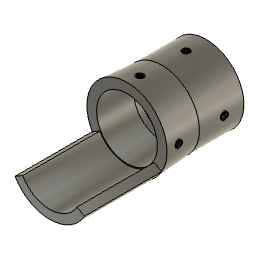
Microscope Holder v3 (Autodesk Fusion 360 design; units mm, degrees)
Autodesk Fusion 360 part; units mm, degrees
sketch "Sketch1" plane through (0, 0, 0) normal (0, 1, 0) x (1, 0, 0)
  circle A0 centre (0, 0) radius 14.5
  dimension "d1" = 29
  constraint coincident A0.centre origin
  measures "d1" diameter of A0
sketch "Sketch2" plane through (0, 0, 0) normal (0, 0, 1) x (1, 0, 0)
  line L0 (0, 0) -> (0, -18)
  dimension "d2" = 18
  constraint coincident L0.start origin
  constraint vertical L0
  measures "d2" distance of L0.start L0.end
sketch "Sketch3" plane through (0, 0, 0) normal (0, 1, 0) x (1, 0, 0)
  circle A0 through (15.75, 0, -18) (-7.875, 13.6399, -18) (-7.875, -13.6399, -18)
  dimension "d3" = 31.5
sketch "Sketch4" plane through (0, 0, 0) normal (0, 1, 0) x (1, 0, 0)
  circle A0 centre (0, 0) radius 19.5
  circle A1 centre (0, 0) radius 14.5
  dimension "d4" = 39
  dimension "d6" = 29
  constraint coincident A0.centre A1.centre
  constraint concentric A0 A1
  measures "d4" diameter of A0
  measures "d6" diameter of A1
sketch "Sketch5" plane through (0, -18, 0) normal (0, 1, 0) x (1, 0, 0)
  circle A0 centre (0, 0) radius 20.75
  circle A1 centre (0, 0) radius 15.75
  dimension "d5" = 41.5
  dimension "d7" = 31.5
  constraint coincident A0.centre A1.centre
  constraint concentric A0 A1
  measures "d5" diameter of A0
  measures "d7" diameter of A1
loft "Loft1" add profiles "Sketch4", "Sketch5" section 1 section 2
loft "Loft2" cut profiles "Sketch4", "Sketch5" section 1 contours A1 section 2 contours A1
extrude "Extrude1" add sketch "Sketch4" along normal blind 3
extrude "Extrude2" add 1 faces at (17.7067, 3, 1.6891) along direction (0, 1, 0) blind 0.05
sketch "Sketch6" plane through (0, 3.05, 0) normal (0, 1, 0) x (-1, 0, 0)
  circle A0 centre (0, 0) radius 14.5
  circle A1 centre (0, 0) radius 19.5
  circle A2 centre (0, 0) radius 10.775
  circle A3 centre (0, 0) radius 19.5
  dimension "d12" = 21.55
  constraint concentric A0 A2
  constraint concentric A0 A3
  measures "d12" diameter of A2
extrude "Extrude3" add sketch "Sketch6" along normal blind 20 contours A0 | A1 A3
sketch "Sketch7" plane through (0, 0, 0) normal (0, 0, 1) x (1, 0, 0)
  line L0 (0, 30) -> (0, -28)
  constraint vertical L0
hole "Hole1" at (0, 12.8255, 19.5) direction (0, 0, -1) diameter 3.416 depth 20 tip angle 118
thread "Thread1" "ANSI Unified Screw Threads 0.164(#8) 8-32 UNC 2B" major diameter 4.1656 minor diameter 3.4163 pitch 0.7937 angle 60 modelled right hand crest width 0.2341 on face at (1.2982, 11.7157, 13.6163) crest through (1.7082, 12.8255, 19.3016)
hole "Hole2" at (0, -11.0084, 20.2645) direction (0, -0.069278, -0.997597) diameter 3.416 depth 20 tip angle 118
thread "Thread2" "ANSI Unified Screw Threads 0.164(#8) 8-32 UNC 2B" major diameter 4.1656 minor diameter 3.4163 pitch 0.7937 angle 60 modelled right hand crest width 0.2341 on face at (0.105, -9.4229, 18.4871) crest through (1.7082, -11.0221, 20.0665)
sketch "Sketch8" plane through (0, -18, 0) normal (0, -1, 0) x (1, 0, 0)
  circle A0 centre (0, 0) radius 15.75
  circle A1 centre (0, 0) radius 20.75
  line L0 (0, 0) -> (0, -20.75) construction
  line L1 (0, 0) -> (0, -20.75) construction
  arc A2 (0, -16.25) -> (14.0729, -8.125) centre (0, 0) ccw
  line L2 (0, 0) -> (0, -16.25) construction
  line L3 (0, 0) -> (14.0729, -8.125) construction
  arc A3 (-14.0729, -8.125) -> (0, -16.25) centre (0, 0) ccw
  line L4 (0, 0) -> (-14.0729, -8.125) construction
  line L5 (0, 0) -> (0, -16.25) construction
  arc A4 (-17.97, -10.375) -> (0, -20.75) centre (0, 0) ccw
  arc A5 (0, -20.75) -> (17.97, -10.375) centre (0, 0) ccw
  line L6 (17.97, -10.375) -> (14.0729, -8.125)
  line L7 (-14.0729, -8.125) -> (-17.97, -10.375)
  dimension "d27" = 60
  dimension "d28" = 60
  constraint coincident A1 L0.end
  constraint coincident A0.centre A1.centre
  constraint coincident A1 A5.end
  constraint parallel L3 L6
  measures "d27" angle of L2 L3
  measures "d28" angle of L4 L5
extrude "Extrude4" add sketch "Sketch8" along normal blind 40 contours A1 A2 A3 A4 A5 L6 L7
hole "Hole3" at (20.2832, -11.2778, 0) direction (-0.997597, -0.069278, 0) diameter 3.416 depth 20 tip angle 118
thread "Thread3" "ANSI Unified Screw Threads 0.164(#8) 8-32 UNC 2B" major diameter 4.1656 minor diameter 3.4163 pitch 0.7937 angle 60 modelled right hand crest width 0.2341 on face at (18.7422, -13.0949, 0.0831) crest through (19.9669, -9.5875, 0)
hole "Hole4" at (19.5, 13.1678, 0) direction (-1, 0, 0) diameter 3.416 depth 20 tip angle 118
thread "Thread4" "ANSI Unified Screw Threads 0.164(#8) 8-32 UNC 2B" major diameter 4.1656 minor diameter 3.4163 pitch 0.7937 angle 60 modelled right hand crest width 0.2341 on face at (13.6079, 12.1721, -1.3877) crest through (19.3016, 14.876, 0)
